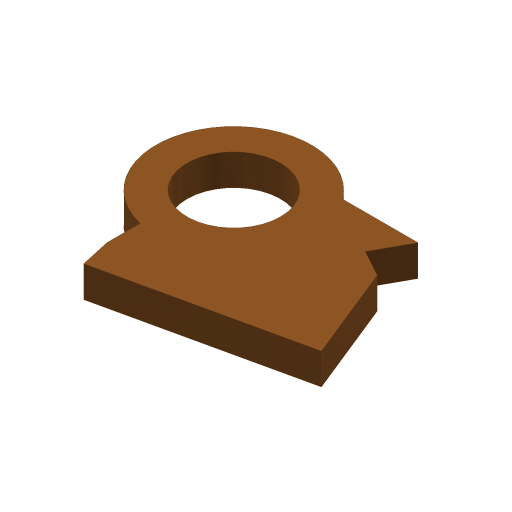
# Autodesk Inventor part: Kontakt
Saved by Autodesk Inventor 2023 (Build 270158000, 158)
## iProperties
Created: 2025-01-25
Part Number: Kontakt
Material: 2.0265 CuZn30(Bronze/weich)
Document SubType Name: Modeling
Designer: abdel
Density: 8.874 g/cm^3
Appearance: Metall - Bronze(poliert)
Author: abdel
Autodesk Inventor part; units mm, degrees
ref_plane "YZ Plane" through (0, 0, 0) normal (1, 0, 0) x (0, 1, 0)
ref_plane "XZ Plane" through (0, 0, 0) normal (0, 1, 0) x (-1, 0, 0)
ref_plane "XY Plane" through (0, 0, 0) normal (0, 0, 1) x (1, 0, 0)
sketch "Skizze1" plane through (0, 0, 0) normal (0, 0, 1) x (1, 0, 0)
  line L0 (-0.1001, 7.9841) -> (4.7481, 7.9841)
  line L1 (5.2519, 4.8576) -> (5.2519, 0)
  line L2 (5.2519, 0) -> (-5.2519, 0)
  line L3 (-5.2519, 0) -> (-5.2519, 0.1317)
  line L4 (0, 14.3325) -> (0, -2.5319) projected
  line L5 (-14.2928, 0) -> (8.5093, 0) projected
  line L6 (4.7481, 7.9841) -> (3.547, 5.7916)
  line L7 (3.547, 5.7916) -> (5.2519, 4.8576)
  arc A0 (-0.1001, 7.9841) -> (-5.2519, 0.1317) centre (-4.112, 5) ccw
  point P0 (0, 0)
  dimension "d34" = 8
  dimension "d36" = 2.5
  dimension "d40" = 10
  dimension "d41" = 61.286
  dimension "d42" = 5.2519
  dimension "d43" = 7.9841
  dimension "d44" = 0.1002
  constraints: 12 end point, 2 parallel, 2 perpendicular, 2 point on circle, 2 point on line, 1 centre point, 1 horizontal, 1 midpoint, 1 tangent
  measures "d34" distance of L0.end L1.end
  measures "d36" distance of L0.end L6.end
  measures "d40" diameter of A0
  measures "d41" angle of L4 L7
  measures "d42" distance between parallel lines of L4 L1
  measures "d43" distance between parallel lines of L0 L5
  measures "d44" distance from line of L0.start L4
extrude "Extrusion2" add sketch "Skizze1" along normal blind 2
sketch "Skizze4" plane through (0, 0, 2) normal (0, 0, 1) x (1, 0, 0)
  arc A0 (-0.1001, 7.9841) -> (-5.2519, 0.1317) centre (-4.112, 5) ccw projected
  point P0 (0, 0)
  constraints: 1 coincident
hole "Bohrung2" at (-4.112, 5, 2) direction (0, 0, -1) diameter 6 end through all
sketch "Skizze5" plane through (-5.2519, 0, 0) normal (0, -1, 0) x (1, 0, 0)
  line L0 (0, 0) -> (10.5038, 0) projected
  line L1 (10.5038, 0) -> (10.5038, 2) projected
  line L2 (0, 2) -> (10.5038, 2) projected
  line L3 (0, 0) -> (0, 2) projected
  point P0 (5.2519, 0)
extrude "Extrusion3" add sketch "Skizze5" along normal blind 2
sketch "Skizze6" plane through (5.2519, 4.8576, 2) normal (1, 0, 0) x (0, 0, -1)
  line L0 (2, 0) -> (2, -6.8576) projected
  line L1 (2, 0) -> (0, 0) projected
  line L2 (0, 0) -> (0, -6.8576) projected
  line L3 (2, -6.8576) -> (0, -6.8576) projected
  point P0 (2, -4.8576)
extrude "Extrusion4" add sketch "Skizze6" along normal blind 2
sketch "Skizze7" plane through (0, 0, 2) normal (0, 0, 1) x (1, 0, 0)
  line L0 (-5.2519, -2) -> (7.2519, -2) projected
  line L1 (7.2519, 4.8576) -> (7.2519, -2) projected
  line L2 (-5.2519, -2) -> (7.2519, 0.7766)
  line L3 (-5.2519, -2) -> (7.5565, -2) construction
  point P0 (0, 0)
  dimension "d56" = 12.52
  constraints: 4 end point, 1 equal length, 1 horizontal, 1 point on line
  measures "d56" angle of L3 L2
extrude "Extrusion5" cut sketch "Skizze7" against normal blind 2
sketch "Skizze8" plane through (-5.2519, -2, 0) normal (0.2168, -0.9762, 0) x (0.9762, 0.2168, 0)
  line L0 (0, 2) -> (12.8083, 2) projected
  line L1 (0, 2) -> (0, 0) projected
  line L2 (12.8083, 0) -> (0, 0) projected
  line L3 (12.8083, 2) -> (12.8083, 0) projected
  point P0 (5.5605, 0)
extrude "Extrusion6" add sketch "Skizze8" along normal blind 1.98
sketch "Skizze9" plane through (0, 0, 2) normal (0, 0, 1) x (1, 0, 0)
  line L0 (7.2519, 4.8576) -> (7.2519, 0.7766) projected
  line L1 (5.2519, 4.8576) -> (7.2519, 4.8576) projected
  line L2 (7.6811, -1.1563) -> (-4.8227, -3.9329) projected
  line L3 (7.2519, 0.7766) -> (7.6811, -1.1563) projected
  line L4 (5.2519, 4.8576) -> (7.6811, -1.1563)
  point P0 (0, 0)
  constraints: 2 end point, 1 point on line
extrude "Extrusion7" cut sketch "Skizze9" against normal blind 2
